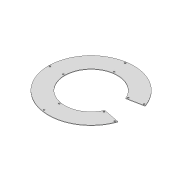
# Autodesk Inventor part: Shelf
Saved by Autodesk Inventor 2021 (Build 250183000, 183)
## iProperties
Created: 2020-07-30
Part Number: Shelf
Material: Generic
Document SubType Name: Modeling
Designer: Dan Wikman
Density: 1 g/cm^3
Appearance: Default
Author: Dan Wikman
Autodesk Inventor part; units mm, degrees
ref_plane "YZ Plane" through (0, 0, 0) normal (1, 0, 0) x (0, 1, 0)
ref_plane "XZ Plane" through (0, 0, 0) normal (0, 1, 0) x (-1, 0, 0)
ref_plane "XY Plane" through (0, 0, 0) normal (0, 0, 1) x (1, 0, 0)
sketch "Sketch1" plane through (0, 0, 0) normal (0, 1, 0) x (-1, 0, 0)
  line L0 (-548.1175, 185.8202) -> (-328.9504, 143.2184)
  line L1 (-547.9214, -184.3469) -> (-328.7026, -141.7351)
  arc A0 (-547.9214, -184.3469) -> (-548.1175, 185.8202) centre (-2.1062, 1.0257) ccw
  arc A1 (-328.7026, -141.7351) -> (-328.9504, 143.2184) centre (-2.1062, 1.0257) ccw
  circle A2 centre (-340.5404, 165.8456) radius 10
  circle A3 centre (-521.3675, 200.9948) radius 10
  line L2 (-296.1915, 1.3356) -> (-698.7298, 1.3356)
  circle A4 centre (-340.5404, -163.1743) radius 10
  circle A5 centre (-521.3675, -198.3235) radius 10
  circle A6 centre (376.435, 0) radius 10
  circle A7 centre (556.435, 0) radius 10
  circle A8 centre (58.8874, 371.8005) radius 10
  circle A9 centre (87.0456, 549.5844) radius 10
  circle A10 centre (58.8874, -371.8005) radius 10
  circle A11 centre (87.0456, -549.5844) radius 10
  point P0 (0, 0)
  dimension "d34" = 1152.87
  dimension "d48" = 712.87
  dimension "d52" = 20
  dimension "d53" = 20
  dimension "d54" = 376.435
  dimension "d55" = 20
  dimension "d56" = 20
  dimension "d58" = 556.435
  dimension "d59" = 20
  dimension "d60" = 376.435
  dimension "d61" = 20
  dimension "d62" = 556.435
  dimension "d65" = 81
  dimension "d69" = 81
  constraints: 12 centre point, 6 end point, 4 point on circle, 2 symmetric about line, 1 coincident, 1 horizontal, 12 other
  measures "d34" diameter of A0
  measures "d48" diameter of A1
  measures "d52" diameter of A2
  measures "d53" distance from line of L0 A2.centre
  measures "d54" distance of A1.centre A2.centre
  measures "d55" diameter of A3
  measures "d56" distance from line of L0 A3.centre
  measures "d58" distance of A0.centre A3.centre
  measures "d59" diameter of A6
  measures "d60" distance of point (0, 0) A6.centre
  measures "d61" diameter of A7
  measures "d62" distance of point (0, 0) A7.centre
extrude "Extrusion1" add sketch "Sketch1" along normal blind 7
body "Solid1"
